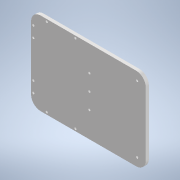
# Autodesk Inventor part: fleet_top
Saved by Autodesk Inventor 2020 (Build 240168000, 168)
## iProperties
Created: 2020-01-06
Part Number: fleet_top
Material: Generic
Document SubType Name: Modeling
Designer: my
Density: 1 g/cm^3
Appearance: Default
Author: my
Autodesk Inventor part; units mm, degrees
ref_plane "YZ Plane" through (0, 0, 0) normal (1, 0, 0) x (0, 1, 0)
ref_plane "XZ Plane" through (0, 0, 0) normal (0, 1, 0) x (-1, 0, 0)
ref_plane "XY Plane" through (0, 0, 0) normal (0, 0, 1) x (1, 0, 0)
sketch "Sketch1" plane through (0, 0, 0) normal (0, 0, 1) x (1, 0, 0)
  line L0 (-75, -65) -> (75, -65)
  line L1 (90, -50) -> (90, 50)
  line L2 (75, 65) -> (-75, 65)
  line L3 (-90, 50) -> (-90, -50)
  line L4 (-90, -65) -> (90, 65) construction
  line L5 (90, -65) -> (-90, 65) construction
  arc A0 (-75, 65) -> (-90, 50) centre (-75, 50) ccw
  arc A1 (-90, -50) -> (-75, -65) centre (-75, -50) ccw
  arc A2 (75, -65) -> (90, -50) centre (75, -50) ccw
  arc A3 (90, 50) -> (75, 65) centre (75, 50) ccw
  point P0 (0, 0)
  dimension "d0" = 130
  dimension "d1" = 180
  dimension "d2" = 15
  dimension "d3" = 15
  constraints: 12 end point, 8 point on circle, 8 point on line, 8 tangent, 4 centre point, 2 equal radius, 2 midpoint, 2 parallel, 1 horizontal, 1 perpendicular
  measures "d0" distance of L5.start L4.end
  measures "d1" distance of L4.end L5.end
  measures "d2" radius of A0
  measures "d3" radius of A1
extrude "Extrusion1" add sketch "Sketch1" along normal blind 5
sketch "Sketch2" plane through (0, 0, 0) normal (0, 0, -1) x (-1, 0, 0)
  circle A0 centre (65.5, 61.5) radius 2 projected
  circle A1 centre (86.5, 46) radius 2 projected
  circle A2 centre (20.5, 61.5) radius 2 projected
  circle A3 centre (86.5, 29) radius 2 projected
  line L0 (12.5, 65) -> (12.5, 57) projected
  line L1 (12.5, 57) -> (75, 57) projected
  arc A4 (82, 50) -> (75, 57) centre (75, 50) ccw projected
  line L2 (82, 50) -> (82, 23) projected
  line L3 (82, 23) -> (90, 23) projected
  line L4 (90, 23) -> (90, 50) projected
  arc A5 (90, 50) -> (75, 65) centre (75, 50) ccw projected
  line L5 (75, 65) -> (12.5, 65) projected
  circle A6 centre (-1.5, -25) radius 2 projected
  circle A7 centre (-1.5, 0) radius 2 projected
  circle A8 centre (-1.5, 25) radius 2 projected
  arc A9 (4.5, 33) -> (2.5, 35) centre (2.5, 33) ccw projected
  line L6 (2.5, 35) -> (-5.5, 35) projected
  arc A10 (-5.5, 35) -> (-7.5, 33) centre (-5.5, 33) ccw projected
  line L7 (-7.5, 33) -> (-7.5, -33) projected
  arc A11 (-7.5, -33) -> (-5.5, -35) centre (-5.5, -33) ccw projected
  line L8 (-5.5, -35) -> (2.5, -35) projected
  arc A12 (2.5, -35) -> (4.5, -33) centre (2.5, -33) ccw projected
  line L9 (4.5, -33) -> (4.5, 33) projected
  circle A13 centre (-76.5, 52) radius 2 projected
  circle A14 centre (-76.5, 52) radius 7.5 projected
  circle A15 centre (-76.5, -52) radius 2 projected
  circle A16 centre (20.5, -61.5) radius 2 projected
  circle A17 centre (65.5, -61.5) radius 2 projected
  circle A18 centre (86.5, -29) radius 2 projected
  circle A19 centre (86.5, -46) radius 2 projected
  line L10 (12.5, -57) -> (12.5, -65) projected
  line L11 (12.5, -65) -> (75, -65) projected
  arc A20 (75, -65) -> (90, -50) centre (75, -50) ccw projected
  line L12 (90, -50) -> (90, -23) projected
  line L13 (90, -23) -> (82, -23) projected
  line L14 (82, -23) -> (82, -50) projected
  arc A21 (75, -57) -> (82, -50) centre (75, -50) ccw projected
  line L15 (75, -57) -> (12.5, -57) projected
  point P0 (0, 0)
hole "Hole1" at (-86.5, -29, 0) at (-86.5, -46, 0) at (-65.5, -61.5, 0) at (-20.5, -61.5, 0) at (1.5, -25, 0) at (1.5, 0, 0) at (1.5, 25, 0) at (76.5, -52, 0) at (76.5, 52, 0) at (-20.5, 61.5, 0) at (-65.5, 61.5, 0) at (-86.5, 46, 0) at (-86.5, 29, 0) direction (0, 0, 1) diameter 3.4 end through all countersink diameter 6.3 countersink angle 90 clearance for "Countersunk Flat Head Screw ISO 2009/7046" size "M3" standard "ISO"
body "Solid1"
